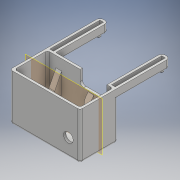
# Autodesk Inventor part: switchcase2
Saved by Autodesk Inventor 2018 (Build 220112000, 112)
## iProperties
Created: 2017-12-19
Part Number: switchcase2
Material: Generic
Document SubType Name: Modeling
Designer: ragna
Density: 1 g/cm^3
Appearance: Default
Author: ragna
Autodesk Inventor part; units mm, degrees
ref_plane "YZ Plane" through (0, 0, 0) normal (1, 0, 0) x (0, 1, 0)
ref_plane "XZ Plane" through (0, 0, 0) normal (0, 1, 0) x (-1, 0, 0)
sketch "Sketch1" plane through (0, 0, 0) normal (0, 0, 1) x (1, 0, 0)
  line L0 (-60.2, 89.46) -> (-52.7, 89.46) projected
  line L1 (-60.2, 0) -> (-60.2, 89.46) projected
  line L2 (-52.7, 0) -> (-60.2, 0) projected
  line L3 (-52.7, 0) -> (-52.7, 89.46) projected
  circle A0 centre (-56.45, 5.3) radius 1.5 projected
  line L4 (-7.5, 89.46) -> (0, 89.46) projected
  line L5 (-7.5, 0) -> (-7.5, 89.46) projected
  line L6 (0, 0) -> (-7.5, 0) projected
  line L7 (0, 0) -> (0, 89.46) projected
  circle A1 centre (-3.75, 6.3) radius 1.5 projected
  line L8 (-0.2, 89.26) -> (-7.3, 89.26)
  line L9 (-7.3, 89.26) -> (-7.3, 0.2)
  line L10 (-7.3, 0.2) -> (-0.2, 0.2)
  line L11 (-0.2, 0.2) -> (-0.2, 89.26)
  line L12 (-52.9, 89.26) -> (-60, 89.26)
  line L13 (-60, 89.26) -> (-60, 0.2)
  line L14 (-60, 0.2) -> (-52.9, 0.2)
  line L15 (-52.9, 0.2) -> (-52.9, 89.26)
  line L16 (-52.9, 10) -> (-60, 10)
  line L17 (-0.2, 10) -> (-7.3, 10)
  dimension "d0" = 0.2
  dimension "d1" = 0.2
  dimension "d2" = 10
  dimension "d3" = 10
  constraints: 20 end point, 4 point on line, 2 perpendicular, 6 other
  measures "d0" distance between parallel lines of L7 L11
  measures "d1" distance between parallel lines of L3 L15
  measures "d2" distance between parallel lines of L2 L16
  measures "d3" distance between parallel lines of L6 L17
ref_plane "Work Plane1" through (0, 0, 6.9) normal (0, 0, 1) x (1, 0, 0)
extrude "Extrusion1" add sketch "Sketch1" along normal up to surface (6.9 mm away) contours L11 L10 L9 L17 | L15 L14 L13 L16
sketch "Sketch2" plane through (-7.3, 0.2, 6.9) normal (0, 0, 1) x (1, 0, 0)
  circle A0 centre (3.55, 6.1) radius 1.5 projected
  circle A1 centre (-49.15, 5.1) radius 1.5 projected
  point P0 (7.3, -0.2)
extrude "Extrusion2" add sketch "Sketch2" against normal blind 10
sketch "Sketch3" plane through (-7.3, 0.2, 0) normal (0, -1, 0) x (1, 0, 0)
  line L0 (7.1, 6.9) -> (0, 6.9) projected
  line L1 (0, 0) -> (0, 6.9) projected
  line L2 (0, 0) -> (7.1, 0) projected
  line L3 (7.1, 0) -> (7.1, 6.9) projected
  line L4 (-45.6, 6.9) -> (-52.7, 6.9) projected
  line L5 (-52.7, 0) -> (-52.7, 6.9) projected
  line L6 (-52.7, 0) -> (-45.6, 0) projected
  line L7 (-45.6, 0) -> (-45.6, 6.9) projected
  point P0 (7.3, 0)
extrude "Extrusion3" add sketch "Sketch3" along normal blind 35
sketch "Sketch4" plane through (-7.3, 10, 6.9) normal (0, 0, 1) x (1, 0, 0)
  line L0 (7.1, -44.8) -> (0, -44.8) projected
  line L1 (-45.6, -44.8) -> (-52.7, -44.8) projected
  line L2 (7.1, 0) -> (7.1, -44.8) projected
  line L3 (7.1, -44.8) -> (-52.7, -44.8)
  line L4 (-52.7, -44.8) -> (-52.7, -76.8)
  line L5 (-52.7, -76.8) -> (7.1, -76.8)
  line L6 (7.1, -76.8) -> (7.1, -44.8)
  line L7 (5.1, -74.8) -> (-50.7, -74.8)
  line L8 (-50.7, -74.8) -> (-50.7, -46.8)
  line L9 (-50.7, -46.8) -> (5.1, -46.8)
  line L10 (5.1, -46.8) -> (5.1, -74.8)
  point P0 (7.3, -10)
  dimension "d10" = 32
  dimension "d11" = 2
  constraints: 16 end point, 4 parallel, 2 perpendicular, 1 horizontal, 3 other
  measures "d10" distance of L4.end L3.end
  measures "d11" distance between parallel lines of L5 L7
extrude "Extrusion4" add sketch "Sketch4" against normal blind 38
ref_plane "Work Plane2" through (-58, -50.8, 6.9) normal (0, -1, 0) x (1, 0, 0)
sketch "Sketch5" plane through (-58, -64.8, 6.9) normal (0, 1, 0) x (1, 0, 0)
  circle A0 centre (47.8333, 25.3333) radius 4.1
  line L0 (57.8, 0) -> (57.8, 38) projected
  line L1 (-2, 0) -> (-2, 38) projected
  line L2 (-2, 0) -> (57.8, 0) projected
  line L3 (57.8, 38) -> (-2, 38) projected
  point P0 (58, 6.9)
  dimension "d14" = 8.2
  dimension "d15" = 59.8
  dimension "d16" = 9.9667
  dimension "d17" = 38
  dimension "d18" = 12.6667
  constraints: 1 centre point
  measures "d14" diameter of A0
  measures "d15" distance between parallel lines of L0 L1
  measures "d16" distance from line of L0 A0.centre
  measures "d17" distance between parallel lines of L2 L3
  measures "d18" distance from line of L3 A0.centre
extrude "Extrusion5" cut sketch "Sketch5" against normal blind 38 contours A0
sketch "Sketch6" plane through (-58, -64.8, 6.9) normal (0, 1, 0) x (1, 0, 0)
  line L0 (12.125, 21.15) -> (7.275, 21.15) projected
  line L1 (12.125, 37.1) -> (12.125, 21.15) projected
  line L2 (34.725, 21.15) -> (39.575, 21.15) projected
  line L3 (34.725, 37.1) -> (34.725, 21.15) projected
  line L4 (7.275, 21.15) -> (12.125, 21.15)
  line L5 (12.125, 21.15) -> (12.125, 27.15)
  line L6 (12.125, 27.15) -> (7.275, 27.15)
  line L7 (7.275, 27.15) -> (7.275, 21.15)
  line L8 (39.575, 21.15) -> (34.725, 21.15)
  line L9 (34.725, 21.15) -> (34.725, 27.15)
  line L10 (34.725, 27.15) -> (39.575, 27.15)
  line L11 (39.575, 27.15) -> (39.575, 21.15)
  point P0 (58, 6.9)
  dimension "d21" = 6
  constraints: 16 end point, 4 parallel, 3 point on line, 2 horizontal, 2 perpendicular
  measures "d21" distance of L5.end L4.end
extrude "Extrusion6" add sketch "Sketch6" along normal up to next
sketch "Sketch7" plane through (-23.275, -64.8, -14.25) normal (0, 0, 1) x (1, 0, 0)
  circle A0 centre (2.6, 14) radius 1.05 projected
  circle A1 centre (-25.2, 14) radius 1.05 projected
  point P0 (23.275, 64.8)
extrude "Extrusion7" cut sketch "Sketch7" against normal up to next
sketch "Sketch8" plane through (-7.3, 10, -31.1) normal (0, 0, -1) x (-1, 0, 0)
  line L0 (-5.1, -74.8) -> (-5.1, -46.8) projected
  line L1 (-5.1, -46.8) -> (50.7, -46.8) projected
  line L2 (50.7, -46.8) -> (50.7, -74.8) projected
  line L3 (50.7, -74.8) -> (-5.1, -74.8) projected
  line L4 (52.7, -44.8) -> (-7.1, -44.8) projected
  line L5 (-7.1, -44.8) -> (-7.1, -76.8) projected
  line L6 (-7.1, -76.8) -> (52.7, -76.8) projected
  line L7 (52.7, -76.8) -> (52.7, -44.8) projected
  point P0 (-7.3, -10)
extrude "Extrusion8" add sketch "Sketch8" along normal blind 2 contours L0 L1 L2 L3 | L7 L6 L5 L4
sketch "Sketch9" plane through (-7.3, 10, 6.9) normal (0, 0, 1) x (1, 0, 0)
  line L0 (0, -44.8) -> (0, 0) projected
  line L1 (0, 0) -> (7.1, 0) projected
  line L2 (7.1, 0) -> (7.1, -76.8) projected
  line L3 (-52.7, -76.8) -> (-52.7, 0) projected
  line L4 (-52.7, 0) -> (-45.6, 0) projected
  line L5 (-45.6, 0) -> (-45.6, -44.8) projected
  line L6 (-50.7, -71.8) -> (-50.7, -2)
  line L7 (-50.7, -2) -> (-47.6, -2)
  line L8 (-47.6, -2) -> (-47.6, -44.8)
  line L9 (2, -44.8) -> (2, -2)
  line L10 (2, -2) -> (5.1, -2)
  line L11 (5.1, -2) -> (5.1, -71.8)
  line L12 (-47.6, -44.8) -> (-50.7, -44.8)
  line L13 (-52.7, -44.8) -> (7.1, -44.8) projected
  line L14 (2, -44.8) -> (5.1, -44.8)
  point P0 (7.3, -10)
  dimension "d28" = 2
  dimension "d29" = 2
  constraints: 16 end point, 4 point on line, 4 other
  measures "d28" distance between parallel lines of L3 L6
  measures "d29" distance between parallel lines of L0 L9
extrude "Extrusion9" cut sketch "Sketch9" against normal blind 4.9 contours L9 L10 L11 L13 | L6 L7 L8 L12
chamfer "Chamfer1" distance 12 distance2 7 1 edges at (-20.85, -64.8, -14.25) measured on face at (-27.825, -64.8, -0.15)
chamfer "Chamfer2" distance 12 distance2 7 1 edges at (-48.3, -64.8, -14.25) measured on face at (-42.3833, -64.8, -3.2)
fillet "Fillet1" radius 2 16 edges at (-58, -64.8, -12.1) (-60, -66.8, -13.1) (-60, -50.8, -33.1) (-30.1, -66.8, -33.1) (-0.2, -66.8, -13.1) (-2.2, -36.8, -12.1) (-58, -36.8, -12.1) (-0.2, -34.8, -16.55) (-0.2, -50.8, -33.1) (-30.1, -64.8, -31.1) (-2.2, -50.8, -31.1) (-30.1, -36.8, -31.1) (-58, -50.8, -31.1) (-30.1, -34.8, -33.1) (-60, -34.8, -16.55) (-2.2, -64.8, -12.1)
sketch "Sketch10" plane through (-52.9, -34.8, 6.9) normal (0, 1, 0) x (1, 0, 0)
  line L0 (45.6, 0) -> (0, 0) construction
  line L1 (22.8, 0) -> (22.8, 40) construction
  line L2 (50.7, 40) -> (-5.1, 40) construction
  line L3 (45.6, 0) -> (22.8, 0)
  line L4 (22.8, 0) -> (22.8, 12)
  line L5 (22.8, 12) -> (45.6, 12)
  line L6 (45.6, 12) -> (45.6, 0)
  point P0 (52.9, 6.9)
  dimension "d39" = 12
  constraints: 10 end point, 2 midpoint, 2 parallel, 1 horizontal, 1 perpendicular, 1 point on line
  measures "d39" distance of L3.end L4.end
extrude "Extrusion10" cut sketch "Sketch10" against normal up to next
fillet "Fillet2" radius 1 6 edges at (-56.45, 10, 0) (-60, 5.1, 0) (-52.9, -12.4, 0) (-7.3, -12.4, 0) (-3.75, 10, 0) (-0.2, -13.4, 0)
fillet "Fillet3" radius 3 8 edges at (-53.1929, 9.7071, 0.2929) (-52.9, 10, 3.95) (-59.7071, 9.7071, 0.2929) (-60, 10, 3.95) (-7.0071, 9.7071, 0.2929) (-7.3, 10, 3.95) (-0.4929, 9.7071, 0.2929) (-0.2, 10, 3.95)
fillet "Fillet4" radius 0.5 2 edges at (-57.95, 5.3, -3.1) (-5.25, 6.3, -3.1)
fillet "Fillet5" radius 3 2 edges at (-7.3, -35.8, -5.1) (-30.1, -35.8, -5.1)
chamfer "Chamfer3" distance 12 distance2 6 1 edges at (-48.3, -36.8, -14.25) measured on face at (-27.825, -36.8, -26.15)
chamfer "Chamfer4" distance 8 distance2 6 1 edges at (-20.85, -36.8, -14.25) measured on face at (-27.825, -36.8, -26.15)
sketch "Sketch11" plane through (-23.275, -57.8, -14.25) normal (0, 0, 1) x (1, 0, 0)
  line L0 (-32.725, 19) -> (19.075, 19) projected
  line L1 (-32.725, -5) -> (-32.725, 19) projected
  line L2 (19.075, -5) -> (-32.725, -5) projected
  line L3 (19.075, 19) -> (19.075, -5) projected
  circle A0 centre (2.6, 7) radius 1.05 projected
  line L4 (0, 15) -> (4.85, 15) projected
  line L5 (0, 0) -> (0, 15) projected
  line L6 (4.85, 0) -> (0, 0) projected
  line L7 (4.85, 0) -> (4.85, 15) projected
  line L8 (0, 21) -> (0, 15) projected
  line L9 (0, 15) -> (4.85, 15) projected
  line L10 (4.85, 15) -> (4.85, 21) projected
  line L11 (4.85, 21) -> (0, 21) projected
  line L12 (0, -7) -> (0, 21) projected
  line L13 (0, 10.6865) -> (1.5, 10.6865)
  line L14 (1.5, 10.6865) -> (1.5, 17.6865)
  line L15 (1.5, 17.6865) -> (0, 17.6865)
  line L16 (0, 17.6865) -> (0, 10.6865)
  point P0 (23.275, 57.8)
  dimension "d52" = 1.5
  dimension "d53" = 7
  constraints: 8 end point, 2 parallel, 1 horizontal, 1 perpendicular, 1 point on line
  measures "d52" distance of L15.end L14.end
  measures "d53" distance of L14.end L13.end
extrude "Extrusion11" cut sketch "Sketch11" along normal up to surface (38 mm away) from surface at -16.85 contours L15 L14 L4 L8 | L4 L14 L13 L5
fillet "Fillet6" radius 3 4 edges at (-21.775, -40.1135, -15.459) (-23.275, -40.1135, -15.459) (-21.775, -47.1135, -17.25) (-23.275, -47.1135, -17.25)
sketch "Sketch12" plane through (-7.3, 10, -33.1) normal (0, 0, -1) x (-1, 0, 0)
  line L0 (64.7017, -60.8) -> (-19.3003, -60.8) projected
  line L1 (23.3, -55.8) -> (22.3, -55.8)
  line L2 (22.3, -55.8) -> (22.3, -65.8)
  line L3 (22.3, -65.8) -> (23.3, -65.8)
  line L4 (23.3, -65.8) -> (23.3, -55.8)
  line L5 (50.7, -46.8) -> (50.7, -74.8) projected
  line L6 (-5.1, -74.8) -> (-5.1, -46.8) projected
  line L7 (20.3, -55.8) -> (19.3, -55.8)
  line L8 (19.3, -55.8) -> (19.3, -65.8)
  line L9 (19.3, -65.8) -> (20.3, -65.8)
  line L10 (20.3, -65.8) -> (20.3, -55.8)
  line L11 (17.3, -55.8) -> (16.3, -55.8)
  line L12 (16.3, -55.8) -> (16.3, -65.8)
  line L13 (16.3, -65.8) -> (17.3, -65.8)
  line L14 (17.3, -65.8) -> (17.3, -55.8)
  line L15 (14.3, -55.8) -> (13.3, -55.8)
  line L16 (13.3, -55.8) -> (13.3, -65.8)
  line L17 (13.3, -65.8) -> (14.3, -65.8)
  line L18 (14.3, -65.8) -> (14.3, -55.8)
  line L19 (26.3, -55.8) -> (25.3, -55.8)
  line L20 (25.3, -55.8) -> (25.3, -65.8)
  line L21 (25.3, -65.8) -> (26.3, -65.8)
  line L22 (26.3, -65.8) -> (26.3, -55.8)
  line L23 (23.3, -55.8) -> (22.3, -55.8)
  line L24 (22.3, -55.8) -> (22.3, -65.8)
  line L25 (22.3, -65.8) -> (23.3, -65.8)
  line L26 (23.3, -65.8) -> (23.3, -55.8)
  line L27 (20.3, -55.8) -> (19.3, -55.8)
  line L28 (19.3, -55.8) -> (19.3, -65.8)
  line L29 (19.3, -65.8) -> (20.3, -65.8)
  line L30 (20.3, -65.8) -> (20.3, -55.8)
  line L31 (17.3, -55.8) -> (16.3, -55.8)
  line L32 (16.3, -55.8) -> (16.3, -65.8)
  line L33 (16.3, -65.8) -> (17.3, -65.8)
  line L34 (17.3, -65.8) -> (17.3, -55.8)
  line L35 (29.3, -55.8) -> (28.3, -55.8)
  line L36 (28.3, -55.8) -> (28.3, -65.8)
  line L37 (28.3, -65.8) -> (29.3, -65.8)
  line L38 (29.3, -65.8) -> (29.3, -55.8)
  line L39 (26.3, -55.8) -> (25.3, -55.8)
  line L40 (25.3, -55.8) -> (25.3, -65.8)
  line L41 (25.3, -65.8) -> (26.3, -65.8)
  line L42 (26.3, -65.8) -> (26.3, -55.8)
  line L43 (23.3, -55.8) -> (22.3, -55.8)
  line L44 (22.3, -55.8) -> (22.3, -65.8)
  line L45 (22.3, -65.8) -> (23.3, -65.8)
  line L46 (23.3, -65.8) -> (23.3, -55.8)
  line L47 (20.3, -55.8) -> (19.3, -55.8)
  line L48 (19.3, -55.8) -> (19.3, -65.8)
  line L49 (19.3, -65.8) -> (20.3, -65.8)
  line L50 (20.3, -65.8) -> (20.3, -55.8)
  line L51 (32.3, -55.8) -> (31.3, -55.8)
  line L52 (31.3, -55.8) -> (31.3, -65.8)
  line L53 (31.3, -65.8) -> (32.3, -65.8)
  line L54 (32.3, -65.8) -> (32.3, -55.8)
  line L55 (29.3, -55.8) -> (28.3, -55.8)
  line L56 (28.3, -55.8) -> (28.3, -65.8)
  line L57 (28.3, -65.8) -> (29.3, -65.8)
  line L58 (29.3, -65.8) -> (29.3, -55.8)
  line L59 (26.3, -55.8) -> (25.3, -55.8)
  line L60 (25.3, -55.8) -> (25.3, -65.8)
  line L61 (25.3, -65.8) -> (26.3, -65.8)
  line L62 (26.3, -65.8) -> (26.3, -55.8)
  line L63 (23.3, -55.8) -> (22.3, -55.8)
  line L64 (22.3, -55.8) -> (22.3, -65.8)
  line L65 (22.3, -65.8) -> (23.3, -65.8)
  line L66 (23.3, -65.8) -> (23.3, -55.8)
  point P0 (-7.3, -10)
  dimension "d57" = 1
  dimension "d58" = 10
  dimension "d59" = 5
  dimension "d60" = 27.4
  dimension "d61" = 27.4
  dimension "d64" = 3
  dimension "d67" = 3
  constraints: 128 end point, 3 horizontal, 2 parallel, 1 perpendicular, 120 other
  measures "d57" distance of L3.end L2.end
  measures "d58" distance of L2.end L1.end
  measures "d59" distance between parallel lines of L0 L1
  measures "d60" distance between parallel lines of L5 L4
  measures "d61" distance between parallel lines of L6 L2
  measures "d64" distance of L1.start L7.start
  measures "d67" distance of L1.start L19.start
extrude "Extrusion12" add sketch "Sketch12" along normal blind 0.5
sketch "Sketch13" plane through (-7.3, 10, -33.1) normal (0, 0, -1) x (-1, 0, 0)
  line L0 (64.7017, -60.8) -> (-19.3003, -60.8) projected
  line L1 (32.8, -58) -> (12.8, -58)
  line L2 (12.8, -58) -> (12.8, -58.5)
  line L3 (12.8, -58.5) -> (32.8, -58.5)
  line L4 (32.8, -58.5) -> (32.8, -58)
  line L5 (32.3, -65.8) -> (32.3, -55.8) projected
  arc A0 (32.8647, -66.9032) -> (20.8499, -58) centre (17.2074, -75.4741) ccw
  arc A1 (32.4215, -67.1348) -> (20.7979, -58.5) centre (17.2074, -75.4741) ccw
  line L6 (32.8, -63.6) -> (12.8, -63.6)
  line L7 (12.8, -63.6) -> (12.8, -63.1)
  line L8 (12.8, -63.1) -> (32.8, -63.1)
  line L9 (32.8, -63.1) -> (32.8, -63.6)
  arc A2 (28.3433, -69.2654) -> (20.2793, -63.1) centre (17.2074, -75.4741) ccw
  arc A3 (27.8999, -69.497) -> (20.2175, -63.6) centre (17.2074, -75.4741) ccw
  line L10 (32.8647, -66.9032) -> (32.4215, -67.1348)
  line L11 (28.3433, -69.2654) -> (27.8999, -69.497)
  point P0 (-7.3, -10)
  dimension "d72" = 20
  dimension "d73" = 0.5
  dimension "d74" = 0.5
  dimension "d75" = 2.3
  dimension "d76" = 0.5
  dimension "d77" = 4.6
  dimension "d78" = 0.5
  constraints: 20 end point, 8 point on circle, 4 centre point, 4 point on line, 4 symmetric about line, 2 parallel, 1 collinear, 1 horizontal, 1 perpendicular
  measures "d72" distance of L3.end L2.end
  measures "d73" distance of L2.end L1.end
  measures "d74" distance between parallel lines of L5 L4
  measures "d75" distance between parallel lines of L0 L3
  measures "d76" radial gap between concentric circles of A1 A0
  measures "d77" radial gap between concentric circles of A1 A2
  measures "d78" radial gap between concentric circles of A2 A3
extrude "Extrusion13" add sketch "Sketch13" along normal blind 0.8 contours A0 L8 A1 L0 | L0 A1 L3 A0 | L8 L9 L6 L5 | L5 L6 A0 L8 | L5 L1 L4 L3 | L3 A0 L1 L5 | A0 L6 A1 L8 | L3 L2 L1 A0 | A1 L6 A2 L8 | A0 L10 A1 L6 | A2 L6 L7 L8 | A2 L11 A3 L6
sketch "Sketch14" plane through (-7.3, 10, -33.1) normal (0, 0, -1) x (-1, 0, 0)
  line L0 (64.7017, -60.8) -> (-19.3003, -60.8) projected
  line L1 (-5.1, -46.8) -> (50.7, -46.8) projected
  line L2 (-5.1, -74.8) -> (-5.1, -46.8) projected
  line L3 (50.7, -74.8) -> (-5.1, -74.8) projected
  line L4 (50.7, -46.8) -> (50.7, -74.8) projected
  line L5 (13.3, -63.6) -> (12.8, -63.6) projected
  line L6 (12.8, -63.6) -> (12.8, -63.1) projected
  line L7 (12.8, -63.1) -> (13.3, -63.1) projected
  line L8 (13.3, -63.1) -> (13.3, -58.5) projected
  line L9 (13.3, -58.5) -> (12.8, -58.5) projected
  line L10 (12.8, -58.5) -> (12.8, -58) projected
  line L11 (12.8, -58) -> (13.3, -58) projected
  line L12 (13.3, -58) -> (13.3, -55.8) projected
  line L13 (13.3, -55.8) -> (14.3, -55.8) projected
  line L14 (14.3, -55.8) -> (14.3, -58) projected
  line L15 (14.3, -58) -> (16.3, -58) projected
  line L16 (16.3, -58) -> (16.3, -55.8) projected
  line L17 (16.3, -55.8) -> (17.3, -55.8) projected
  line L18 (17.3, -55.8) -> (17.3, -58) projected
  line L19 (17.3, -58) -> (19.3, -58) projected
  line L20 (19.3, -58) -> (19.3, -55.8) projected
  line L21 (19.3, -55.8) -> (20.3, -55.8) projected
  line L22 (20.3, -55.8) -> (20.3, -58) projected
  line L23 (20.3, -58) -> (22.3, -58) projected
  line L24 (22.3, -58) -> (22.3, -55.8) projected
  line L25 (22.3, -55.8) -> (23.3, -55.8) projected
  line L26 (23.3, -55.8) -> (23.3, -58) projected
  line L27 (23.3, -58) -> (25.3, -58) projected
  line L28 (25.3, -58) -> (25.3, -55.8) projected
  line L29 (25.3, -55.8) -> (26.3, -55.8) projected
  line L30 (26.3, -55.8) -> (26.3, -58) projected
  line L31 (26.3, -58) -> (28.3, -58) projected
  line L32 (28.3, -58) -> (28.3, -55.8) projected
  line L33 (28.3, -55.8) -> (29.3, -55.8) projected
  line L34 (29.3, -55.8) -> (29.3, -58) projected
  line L35 (29.3, -58) -> (31.3, -58) projected
  line L36 (31.3, -58) -> (31.3, -55.8) projected
  line L37 (31.3, -55.8) -> (32.3, -55.8) projected
  line L38 (32.3, -55.8) -> (32.3, -58) projected
  line L39 (32.3, -58) -> (32.8, -58) projected
  line L40 (32.8, -58) -> (32.8, -58.5) projected
  line L41 (32.8, -58.5) -> (32.3, -58.5) projected
  line L42 (32.3, -58.5) -> (32.3, -63.1) projected
  line L43 (32.3, -63.1) -> (32.8, -63.1) projected
  line L44 (32.8, -63.1) -> (32.8, -63.6) projected
  line L45 (32.8, -63.6) -> (32.3, -63.6) projected
  line L46 (32.3, -63.6) -> (32.3, -65.8) projected
  line L47 (32.3, -65.8) -> (32.2082, -65.8) projected
  arc A0 (32.8647, -66.9032) -> (32.2082, -65.8) centre (17.2074, -75.4741) ccw projected
  line L48 (32.8647, -66.9032) -> (32.4215, -67.1348) projected
  arc A1 (32.4215, -67.1348) -> (31.6096, -65.8) centre (17.2074, -75.4741) ccw projected
  line L49 (31.6096, -65.8) -> (31.3, -65.8) projected
  line L50 (31.3, -65.8) -> (31.3, -65.3542) projected
  arc A2 (31.3, -65.3542) -> (29.8572, -63.6) centre (17.2074, -75.4741) ccw projected
  line L51 (29.8572, -63.6) -> (29.3, -63.6) projected
  line L52 (29.3, -63.6) -> (29.3, -65.8) projected
  line L53 (29.3, -65.8) -> (28.3, -65.8) projected
  line L54 (28.3, -65.8) -> (28.3, -63.6) projected
  line L55 (28.3, -63.6) -> (26.3, -63.6) projected
  line L56 (26.3, -63.6) -> (26.3, -65.8) projected
  line L57 (26.3, -65.8) -> (25.512, -65.8) projected
  arc A3 (28.3433, -69.2654) -> (25.512, -65.8) centre (17.2074, -75.4741) ccw projected
  line L58 (28.3433, -69.2654) -> (27.8999, -69.497) projected
  arc A4 (27.8999, -69.497) -> (23.3, -64.847) centre (17.2074, -75.4741) ccw projected
  line L59 (23.3, -64.847) -> (23.3, -65.8) projected
  line L60 (23.3, -65.8) -> (22.3, -65.8) projected
  line L61 (22.3, -65.8) -> (22.3, -64.3331) projected
  arc A5 (22.3, -64.3331) -> (20.3, -63.6212) centre (17.2074, -75.4741) ccw projected
  line L62 (20.3, -63.6212) -> (20.3, -65.8) projected
  line L63 (20.3, -65.8) -> (19.3, -65.8) projected
  line L64 (19.3, -65.8) -> (19.3, -63.6) projected
  line L65 (19.3, -63.6) -> (17.3, -63.6) projected
  line L66 (17.3, -63.6) -> (17.3, -65.8) projected
  line L67 (17.3, -65.8) -> (16.3, -65.8) projected
  line L68 (16.3, -65.8) -> (16.3, -63.6) projected
  line L69 (16.3, -63.6) -> (14.3, -63.6) projected
  line L70 (14.3, -63.6) -> (14.3, -65.8) projected
  line L71 (14.3, -65.8) -> (13.3, -65.8) projected
  line L72 (13.3, -65.8) -> (13.3, -63.6) projected
  line L73 (38.4332, -62.4359) -> (38.4332, -59.46)
  line L74 (38.4332, -59.46) -> (39.0561, -59.46)
  line L75 (39.0561, -59.46) -> (39.0561, -60.5673)
  line L76 (39.0561, -60.5673) -> (43.1441, -60.5673)
  line L77 (43.1441, -60.5673) -> (43.1441, -59.46)
  line L78 (43.1441, -59.46) -> (43.7027, -59.46)
  spline S0 degree 2 poles (43.7027, -59.46) (43.7027, -60.0878) (44.0586, -60.681) (44.553, -60.7206) knots 0 0 0 1 2 2 2
  line L79 (44.553, -60.7206) -> (44.553, -61.3533)
  line L80 (44.553, -61.3533) -> (39.0561, -61.3533)
  line L81 (39.0561, -61.3533) -> (39.0561, -62.4359)
  line L82 (39.0561, -62.4359) -> (38.4332, -62.4359)
  point P0 (-7.3, -10)
  point P1 (41.4931, -60.8244)
  constraints: 1 other
extrude "Extrusion14" add sketch "Sketch14" along normal up to surface (0.5 mm away) contours L79 L80 L81 L82 L73 L0 | L0 L73 L74 L75 L76 L77 L78 S0 L79
equation "\"d16\" = 0.166667 * d15"
equation "\"d18\" = 0.333333 * d17"
equation "\"d60\" = d61"
body "Solid1"
